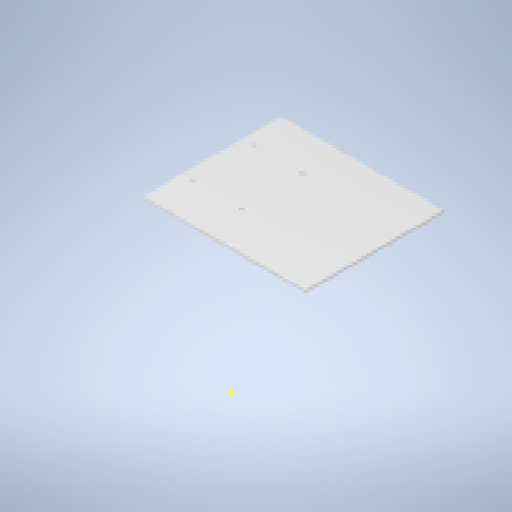
# Autodesk Inventor part: V Rail Gantry
Saved by Autodesk Inventor 2023.2 (Build 272271000, 271)
## iProperties
Created: 2023-02-14
Part Number: V Rail Gantry
Material: Aluminum 6061
Document SubType Name: Modeling
Designer: dmargari
Density: 2.7 g/cm^3
Appearance: Aluminum - Flat
Author: dmargari
Autodesk Inventor part; units mm, degrees
ref_plane "YZ Plane" through (0, 0, 0) normal (1, 0, 0) x (0, 1, 0)
ref_plane "XZ Plane" through (0, 0, 0) normal (0, 1, 0) x (-1, 0, 0)
ref_plane "XY Plane" through (0, 0, 0) normal (0, 0, 1) x (1, 0, 0)
sketch "Sketch1" plane through (0, 0, 0) normal (0, 1, 0) x (-1, 0, 0)
  line L0 (263.2333, -205.0309) -> (63.2333, -205.0309)
  line L1 (63.2333, -205.0309) -> (63.2333, -365.0309)
  line L2 (63.2333, -365.0309) -> (263.2333, -365.0309)
  line L3 (263.2333, -260.0309) -> (263.2333, -205.0309)
  line L4 (249.5333, -205.0309) -> (249.5333, -365.0309) construction
  line L5 (313.2333, -260.0309) -> (63.2333, -260.0309) construction
  line L6 (313.2333, -285.0309) -> (63.2333, -285.0309) construction
  line L7 (249.5333, -365.0309) -> (249.5333, -205.0309) construction
  line L8 (313.2333, -310.0309) -> (63.2333, -310.0309) construction
  line L9 (189.0333, -205.0309) -> (189.0333, -365.0309) construction
  circle A0 centre (249.5333, -260.0309) radius 2.55
  circle A1 centre (249.5333, -310.0309) radius 2.55
  circle A2 centre (189.0333, -260.0309) radius 2.55
  circle A3 centre (189.0333, -310.0309) radius 3.55
  line L10 (219.2833, -205.0309) -> (219.2833, -365.0309) construction
  circle A4 centre (219.2833, -285.0309) radius 1
  line L11 (263.2333, -205.0309) -> (313.2333, -205.0309)
  line L12 (313.2333, -205.0309) -> (313.2333, -365.0309)
  line L13 (313.2333, -365.0309) -> (263.2333, -365.0309)
  line L14 (313.2333, -230.0309) -> (63.2333, -230.0309) construction
  line L15 (313.2333, -340.0309) -> (63.2333, -340.0309) construction
  line L16 (313.2333, -214.7809) -> (270.7929, -214.7809) construction
  circle A5 centre (288.2333, -214.7809) radius 2.55
  line L17 (275.2333, -205.0309) -> (275.2333, -242.3907) construction
  circle A6 centre (288.2333, -245.2809) radius 2.55
  circle A7 centre (262.2333, -214.7809) radius 2.55
  circle A8 centre (262.2333, -245.2809) radius 2.55
  circle A9 centre (288.2333, -355.2809) radius 2.55
  circle A10 centre (288.2333, -324.7809) radius 2.55
  circle A11 centre (262.2333, -355.2809) radius 2.55
  circle A12 centre (262.2333, -324.7809) radius 2.55
  line L18 (213.2333, -205.0309) -> (213.2333, -365.0309) construction
  circle A13 centre (138.2333, -214.7809) radius 2.55
  circle A14 centre (138.2333, -245.2809) radius 2.55
  circle A15 centre (164.2333, -214.7809) radius 2.55
  circle A16 centre (164.2333, -245.2809) radius 2.55
  circle A17 centre (138.2333, -355.2809) radius 2.55
  circle A18 centre (138.2333, -324.7809) radius 2.55
  circle A19 centre (164.2333, -324.7809) radius 2.55
  circle A20 centre (164.2333, -355.2809) radius 2.55
  point P0 (0, 0)
  point P1 (263.2333, -310.0309)
  dimension "d2" = 13.7
  dimension "d4" = 60.5
  dimension "d5" = 5.1
  dimension "d6" = 5.1
  dimension "d7" = 5.1
  dimension "d8" = 7.1
  dimension "d11" = 2
  dimension "d15" = 50
  dimension "d17" = 50
  dimension "d18" = 25
  dimension "d19" = 15.25
  dimension "d20" = 5.1
  dimension "d21" = 13
  dimension "d22" = 25
  dimension "d23" = 160
  dimension "d24" = 75
  constraints: 38 end point, 26 point on line, 21 centre point, 21 symmetric about line, 10 perpendicular, 3 midpoint, 2 horizontal, 2 parallel, 1 vertical, 16 other
  measures "d2" distance between parallel lines of L3 L4
  measures "d4" distance between parallel lines of L4 L9
  measures "d5" diameter of A0
  measures "d6" diameter of A1
  measures "d7" diameter of A2
  measures "d8" diameter of A3
  measures "d11" diameter of A4
  measures "d15" distance between parallel lines of L8 L5
  measures "d17" distance of L0.start L11.end
  measures "d18" distance between parallel lines of L14 L11
  measures "d19" distance between parallel lines of L14 L16
  measures "d20" diameter of A5
  measures "d21" distance from line of L17 A5.centre
  measures "d22" distance from line of L12 A5.centre
  measures "d23" distance between parallel lines of L2 L0
  measures "d24" distance from line of A5.centre L18
extrude "Extrusion1" add sketch "Sketch1" along normal blind 3 contours L11 L12 L13 L2 L1 L0 | A8 L3 | L3 A8 | A7 L3 | L3 A7 | A4 | A5 | A6 | A9 | A10 | A11 | A12 | A13 | A14 | A15 | A16 | A17 | A18 | A19 | A20
sketch "Sketch2" plane through (0, 3, 0) normal (0, 1, 0) x (1, 0, 0)
  point P0 (0, 0)
extrude "Extrusion2" cut sketch "Sketch1" along normal through all contours A4
extrude "Extrusion3" cut sketch "Sketch1" along normal through all contours A8 L3 | L3 A8 | A7 L3 | L3 A7 | A5 | A6 | A9 | A10 | A11 | A12 | A13 | A14 | A15 | A16 | A17 | A18 | A19 | A20
body "Solid1"
